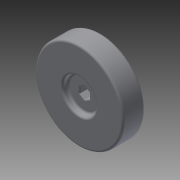
# Autodesk Inventor part: BallShooterWheel000105
Saved by Autodesk Inventor 2015 (Build 190159000, 159)
## iProperties
Created: 2015-05-11
Part Number: BallShooterWheel000105
Material: Generic
Document SubType Name: Modeling
Designer: Caitlynn
Density: 1 g/cm^3
Appearance: Default
Author: Caitlynn
Autodesk Inventor part; units mm, degrees
ref_plane "YZ Plane" through (0, 0, 0) normal (1, 0, 0) x (0, 1, 0)
ref_plane "XZ Plane" through (0, 0, 0) normal (0, 1, 0) x (-1, 0, 0)
ref_plane "XY Plane" through (0, 0, 0) normal (0, 0, 1) x (1, 0, 0)
sketch "Sketch1" plane through (0, 0, 0) normal (0, 0, 1) x (1, 0, 0)
  circle A0 centre (0, 0) radius 25.4
  dimension "d0" = 50.8
  constraints: 1 centre point, 1 coincident
  measures "d0" diameter of A0
extrude "Extrusion1" add sketch "Sketch1" along normal blind 12.7
sketch "Sketch2" plane through (0, 0, 12.7) normal (0, 0, 1) x (1, 0, 0)
  line L0 (0, 3.1852) -> (2.7584, 1.5926)
  line L1 (2.7584, 1.5926) -> (2.7584, -1.5926)
  line L2 (2.7584, -1.5926) -> (0, -3.1852)
  line L3 (0, -3.1852) -> (-2.7584, -1.5926)
  line L4 (-2.7584, -1.5926) -> (-2.7584, 1.5926)
  line L5 (-2.7584, 1.5926) -> (0, 3.1852)
  point P0 (0, 0)
  point P1 (0, 0)
  dimension "d3" = 3.1852
  constraints: 12 end point, 1 coincident, 13 other
  measures "d3" distance of L0.end L1.end
extrude "Extrusion2" cut sketch "Sketch2" against normal through all
sketch "Sketch3" plane through (0, 0, 12.7) normal (0, 0, 1) x (1, 0, 0)
  circle A0 centre (0, 0) radius 9.525
  dimension "d6" = 19.05
  constraints: 1 centre point, 1 coincident
  measures "d6" diameter of A0
extrude "Extrusion3" cut sketch "Sketch3" against normal blind 3.175
fillet "Fillet1" radius 0.762 6 edges at (-1.3792, 2.3889, 9.525) (-2.7584, 0, 9.525) (-1.3792, -2.3889, 9.525) (1.3792, -2.3889, 9.525) (2.7584, 0, 9.525) (1.3792, 2.3889, 9.525)
fillet "Fillet2" radius 0.762 6 edges at (-1.3792, -2.3889, 0) (-2.7584, 0, 0) (-1.3792, 2.3889, 0) (1.3792, 2.3889, 0) (2.7584, 0, 0) (1.3792, -2.3889, 0)
fillet "Fillet3" radius 1.27 4 edges at (-25.4, 0, 12.7) (-25.4, 0, 0) (-9.525, 0, 12.7) (-9.525, 0, 9.525)
body "Solid1"
